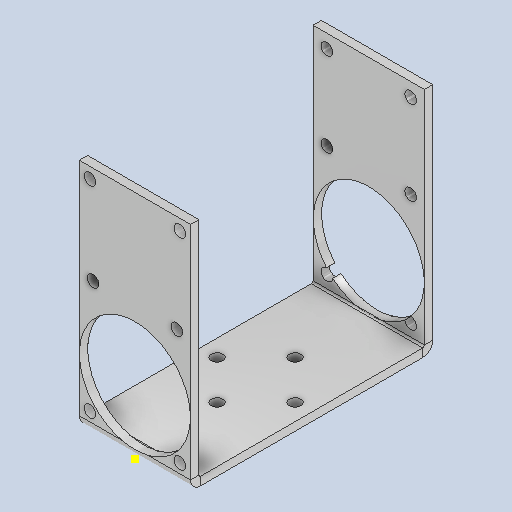
# Autodesk Inventor part: axis_19_top_frame
Saved by Autodesk Inventor 2025.2 (Build 292293000, 293)
## iProperties
Created: 2025-05-06
Part Number: axis_19_top_frame
Material: Aluminum 6061-AHC
Document SubType Name: Sheet Metal
Designer: LG
Density: 2.7 g/cm^3
Sheet Metal Rule: Default_mm
Appearance: Aluminum - Dark
Author: LG
Autodesk Inventor part; units mm, degrees
ref_plane "YZ Plane" through (0, 0, 0) normal (1, 0, 0) x (0, 1, 0)
ref_plane "XZ Plane" through (0, 0, 0) normal (0, 1, 0) x (-1, 0, 0)
ref_plane "XY Plane" through (0, 0, 0) normal (0, 0, 1) x (1, 0, 0)
sketch "Sketch1" plane through (0, 0, 0) normal (0, 1, 0) x (-1, 0, 0)
  line L0 (-10, 20.25) -> (10, 20.25)
  line L1 (10, 20.25) -> (10, -20.25)
  line L2 (10, -20.25) -> (-10, -20.25)
  line L3 (-10, -20.25) -> (-10, 20.25)
  line L4 (-10, 20.25) -> (10, -20.25) construction
  line L5 (10, 20.25) -> (-10, -20.25) construction
  point P0 (0, 0)
  dimension "d0" = 40.5
  dimension "d1" = 20
  measures "d0" distance of L0.end L1.end
  measures "d1" distance of L1.end L2.end
extrude "Plate1" add sketch "Sketch1" along normal blind 1.5
sketch "Sketch2" plane through (-10, 0, -21.75) normal (0, 0, 1) x (1, 0, 0)
  line L0 (20, 0) -> (0, 0)
  line L1 (0, 0) -> (0, 41.55)
  line L2 (0, 41.55) -> (20, 41.55)
  line L3 (20, 41.55) -> (20, 0)
  constraints: 8 end point
edge flange "Flange1" height 41.55 angle 90 thickness 1.5 bend radius 0.31 thickness toward (0, 0, 1) relief straight relief width 1.5 relief depth 0.75 corner gap 0.31 corner form 0 edges at (0, 1.5, -20.25) (0, 1.5, 20.25) wall of the first edge with corners at (10, 0, -21.75) (-10, 0, -21.75) (-10, 41.55, -21.75) (10, 41.55, -21.75)
bend "Bend1"
corner "Corner1"
sketch "Sketch3" plane through (0, 1.5, 0) normal (0, 1, 0) x (1, 0, 0)
  circle A0 centre (7, 0) radius 0.7835 projected
  circle A1 centre (0, -7) radius 0.7835 projected
  circle A2 centre (-7, 0) radius 0.7835 projected
  circle A3 centre (0, 7) radius 0.7835 projected
  point P0 (0, 0)
hole "Hole1" at (0, 1.5, 7) at (7, 1.5, 0) at (-7, 1.5, 0) at (0, 1.5, -7) direction (0, -1, 0) diameter 2.1 depth 1.5
sketch "Sketch4" plane through (-10, 41.55, -20.25) normal (0, 0, 1) x (1, 0, 0)
  point P0 (10, -41.55)
sketch "Sketch5" plane through (-10, 41.55, -20.25) normal (0, 0, 1) x (1, 0, 0)
  point P0 (10, -41.55)
sketch "Sketch6" plane through (-10, 41.55, 21.75) normal (0, 0, 1) x (1, 0, 0)
  circle A0 centre (18.07, -1.95) radius 1.05
  circle A1 centre (17.525, -17.55) radius 0.7835
  circle A2 centre (1.93, -1.95) radius 1.05
  circle A3 centre (2.475, -17.55) radius 0.7835
  circle A4 centre (18.07, -38.05) radius 1.05
  circle A5 centre (1.93, -38.05) radius 1.05
  point P0 (10, -41.55)
  constraints: 6 centre point, 12 other
hole "Hole2" at (8.07, 39.6, 21.75) at (7.525, 24, 21.75) at (8.07, 3.5, 21.75) at (-8.07, 3.5, 21.75) at (-7.525, 24, 21.75) at (-8.07, 39.6, 21.75) direction (0, 0, -1) diameter 2.1 depth 1.5
sketch "Sketch7" plane through (-10, 41.55, 21.75) normal (0, 0, 1) x (1, 0, 0)
  circle A0 centre (10, -30.05) radius 6
  point P0 (10, -41.55)
  constraints: 1 centre point, 2 other
extrude "Cut1" cut sketch "Sketch7" against normal blind 1.5
sketch "Sketch8" plane through (10, 41.55, -21.75) normal (0, 0, -1) x (-1, 0, 0)
  circle A0 centre (2.475, -37.55) radius 1.05
  circle A1 centre (17.525, -37.55) radius 1.05
  circle A2 centre (2.475, -17.55) radius 1.05
  circle A3 centre (17.525, -17.55) radius 1.05
  circle A4 centre (2.475, -2.45) radius 1.05
  circle A5 centre (17.525, -2.45) radius 1.05
  point P0 (10, -41.55)
  constraints: 6 centre point, 12 other
hole "Hole3" at (7.525, 4, -21.75) at (-7.525, 4, -21.75) at (-7.525, 24, -21.75) at (7.525, 24, -21.75) at (7.525, 39.1, -21.75) at (-7.525, 39.1, -21.75) direction (0, 0, 1) diameter 2.1 depth 1.5
sketch "Sketch9" plane through (10, 41.55, -21.75) normal (0, 0, -1) x (-1, 0, 0)
  circle A0 centre (10, -30.05) radius 6
  point P0 (10, -41.55)
  constraints: 1 centre point, 2 other
extrude "Cut2" cut sketch "Sketch9" against normal blind 1.5
sketch "Sketch11" plane through (-10, 41.55, 21.75) normal (0, 0, 1) x (1, 0, 0)
  point P0 (10, -41.55)
sketch "Sketch12" plane through (-10, 41.55, 21.75) normal (0, 0, 1) x (1, 0, 0)
  circle A0 centre (10, -30.05) radius 6.5
  circle A1 centre (10, -30.05) radius 6 projected
  point P0 (10, -41.55)
  dimension "d38" = 13
  constraints: 1 centre point, 1 concentric
  measures "d38" diameter of A0
extrude "Cut3" cut sketch "Sketch12" against normal blind 1.5 contours A0 | A1
sketch "Sketch13" plane through (10, 41.55, -21.75) normal (0, 0, -1) x (-1, 0, 0)
  circle A0 centre (10, -30.05) radius 6.5
  circle A1 centre (10, -30.05) radius 6 projected
  point P0 (10, -41.55)
  dimension "d41" = 13
  constraints: 1 centre point, 1 concentric
  measures "d41" diameter of A0
extrude "Cut4" cut sketch "Sketch13" against normal blind 1.5 contours A0 | A1
sketch "Sketch14" plane through (10, 41.55, -21.75) normal (0, 0, -1) x (-1, 0, 0)
  circle A0 centre (10, -30.05) radius 9.96
  point P0 (10, -41.55)
  constraints: 1 centre point, 2 other
extrude "Cut5" cut sketch "Sketch14" against normal blind 1.5
sketch "Sketch15" plane through (-10, 41.55, 21.75) normal (0, 0, 1) x (1, 0, 0)
  circle A0 centre (10, -30.05) radius 9.96
  point P0 (10, -41.55)
  constraints: 1 centre point, 2 other
extrude "Cut6" cut sketch "Sketch15" against normal blind 1.5
equation "\"d18\" = Thickness"
equation "\"d25\" = Thickness"
equation "\"d27\" = Thickness"
equation "\"d34\" = Thickness"
equation "\"d36\" = Thickness"
equation "\"d39\" = Thickness"
equation "\"d42\" = Thickness"
equation "\"d44\" = Thickness"
equation "\"d46\" = Thickness"
equation "\"d2\" = Thickness"
equation "\"d3\" = BendReliefWidth"
equation "\"d4\" = BendReliefDepth"
equation "\"d5\" = MinimumRemnant"
equation "\"d6\" = TransitionRadius"
equation "\"d9\" = BendRadius"
equation "\"d10\" = CornerReliefSize"
equation "\"d11\" = GapSize"
equation "\"d12\" = JacobiRadiusSize"
equation "\"BendReliefWidth\" = Thickness"
equation "\"BendReliefDepth\" = 0.5 * Thickness"
equation "\"CornerReliefSize\" = 4 * Thickness"
equation "\"MinimumRemnant\" = 2 * Thickness"
equation "\"TransitionRadius\" = BendRadius"
equation "\"JacobiRadiusSize\" = BendRadius"
equation "\"GapSize\" = Thickness"
equation "\"Thickness\" = 1.5"
equation "\"BendRadius\" = 0.31"
body "Solid1"
